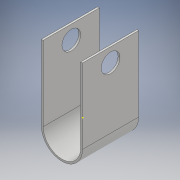
# Autodesk Inventor part: Joiner
Saved by Autodesk Inventor 2018 (Build 220112000, 112)
## iProperties
Created: 2019-06-02
Part Number: Joiner
Material: Generic
Document SubType Name: Modeling
Designer: dell
Density: 1 g/cm^3
Appearance: Default
Author: dell
Autodesk Inventor part; units mm, degrees
ref_plane "YZ Plane" through (0, 0, 0) normal (1, 0, 0) x (0, 1, 0)
ref_plane "XZ Plane" through (0, 0, 0) normal (0, 1, 0) x (-1, 0, 0)
ref_plane "XY Plane" through (0, 0, 0) normal (0, 0, 1) x (1, 0, 0)
sketch "Sketch1" plane through (0, 0, 0) normal (0, 1, 0) x (-1, 0, 0)
  line L0 (0, 14.7497) -> (0, -14.7497) construction
  line L1 (-11, 25.2503) -> (-11, -14.7497)
  line L2 (11, -14.7497) -> (11, 25.2503)
  arc A0 (-11, -14.7497) -> (11, -14.7497) centre (0, -14.7497) ccw
  line L3 (0, 14.7497) -> (0, -14.7497) construction
  line L4 (-10, 25.2503) -> (-10, -14.7497)
  line L5 (10, -14.7497) -> (10, 25.2503)
  arc A1 (-10, -14.7497) -> (10, -14.7497) centre (0, -14.7497) ccw
  line L6 (11, 25.2503) -> (10, 25.2503)
  line L7 (-10, 25.2503) -> (-11, 25.2503)
  point P0 (0, 0)
  dimension "d0" = 22
  dimension "d1" = 20
  dimension "d7" = 40
  dimension "d8" = 40
  constraints: 20 end point, 4 point on circle, 4 tangent, 3 equal length, 2 centre point, 2 horizontal, 2 midpoint, 1 vertical
  measures "d0" diameter of A0
  measures "d1" diameter of A1
  measures "d7" distance of L2.start L2.end
  measures "d8" distance of L1.start L1.end
extrude "Extrusion1" add sketch "Sketch1" along normal blind 30
sketch "Sketch2" plane through (11, 0, 25.2503) normal (1, 0, 0) x (0, 0, -1)
  point P0 (25.2503, 0)
sketch "Sketch3" plane through (11, 0, 25.2503) normal (1, 0, 0) x (0, 0, -1)
  point P0 (25.2503, 0)
sketch "Sketch4" plane through (11, 0, 25.2503) normal (1, 0, 0) x (0, 0, -1)
  line L0 (0, 0) -> (40, 0) projected
  line L1 (40, 0) -> (40, 30) projected
  line L2 (0, 30) -> (40, 30) projected
  line L3 (0, 0) -> (0, 30) projected
  circle A0 centre (7.3749, 15) radius 5
  point P0 (25.2503, 0)
  dimension "d4" = 10
  constraints: 1 centre point
  measures "d4" diameter of A0
extrude "Extrusion2" cut sketch "Sketch4" against normal through all contours A0
body "Solid1"
